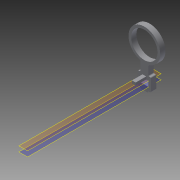
# Autodesk Inventor part: soporte-sujeccion-botella
Saved by Autodesk Inventor 2015 SP1 (Build 190203100, 203)
## iProperties
Created: 2015-07-19
Part Number: soporte-sujeccion-botella
Material: Genérico
Document SubType Name: Modeling
Designer: Javier
Density: 1 g/cm^3
Appearance: Valor por defecto
Author: Javier
Autodesk Inventor part; units mm, degrees
ref_plane "YZ Plane" through (0, 0, 0) normal (1, 0, 0) x (0, 1, 0)
ref_plane "XZ Plane" through (0, 0, 0) normal (0, 1, 0) x (-1, 0, 0)
ref_plane "XY Plane" through (0, 0, 0) normal (0, 0, 1) x (1, 0, 0)
ref_plane "Plano de trabajo1" through (0, 0, 0) normal (0, 0, 1) x (1, 0, 0)
sketch "Boceto1" plane through (0, 0, 0) normal (0, 0, 1) x (1, 0, 0)
  line L0 (9.5, 30) -> (9.5, 0) projected
  line L1 (9.5, 0) -> (15, 0) projected
  line L2 (15, 0) -> (15, 230) projected
  line L3 (0, 230) -> (15, 230) projected
  line L4 (0, 0) -> (0, 230) projected
  line L5 (0, 0) -> (5.5, 0) projected
  line L6 (5.5, 0) -> (5.5, 30) projected
  line L7 (9.5, 30) -> (5.5, 30) projected
  circle A0 centre (7.5, 223) radius 2 projected
  circle A1 centre (7.5, 213) radius 2 projected
  line L8 (0, 218) -> (15, 218)
  line L9 (15, 218) -> (15, 228)
  line L10 (15, 228) -> (0, 228)
  line L11 (0, 228) -> (0, 218)
  line L12 (0, 218) -> (15, 228) construction
  line L13 (15, 218) -> (0, 228) construction
  dimension "d0" = 10
  constraints: 12 end point, 2 midpoint, 2 parallel, 1 horizontal, 1 perpendicular, 1 point on line
  measures "d0" distance of L9.end L8.end
extrude "Extrusión1" add sketch "Boceto1" along normal blind 30 contours L8 L4 L10 L2 | A0
ref_plane "Plano de trabajo2" through (15, 0, -10) normal (0, 0, -1) x (-1, 0, 0)
sketch "Boceto2" plane through (15, 0, -10) normal (0, 0, -1) x (-1, 0, 0)
  line L0 (0, 228) -> (15, 228) projected
  line L1 (15, 228) -> (15, 218) projected
  line L2 (15, 218) -> (0, 218) projected
  line L3 (0, 218) -> (0, 228) projected
  circle A0 centre (7.5, 223) radius 2 projected
  point P0 (15, 0)
extrude "Extrusión2" add sketch "Boceto2" along normal blind 10
sketch "Boceto3" plane through (0, 218, 0) normal (0, -1, 0) x (1, 0, 0)
  line L0 (0, 0) -> (15, 0) projected
  line L1 (15, 0) -> (15, 30) projected
  line L2 (0, 30) -> (15, 30) projected
  line L3 (0, 0) -> (0, 30) projected
  line L4 (0, 0) -> (7.5, 0)
  line L5 (15, 0) -> (0, 0) projected
  line L6 (7.5, 0) -> (7.5, 2.5)
  line L7 (4, 5) -> (11, 5)
  line L8 (11, 5) -> (11, 0)
  line L9 (11, 0) -> (4, 0)
  line L10 (4, 0) -> (4, 5)
  line L11 (4, 5) -> (11, 0) construction
  line L12 (11, 5) -> (4, 0) construction
  dimension "d5" = 2.5
  dimension "d6" = 7
  dimension "d7" = 5
  constraints: 16 end point, 3 midpoint, 2 parallel, 2 perpendicular, 1 horizontal
  measures "d5" distance of L4.end L6.end
  measures "d6" distance of L8.end L9.end
  measures "d7" distance of L7.end L8.end
extrude "Extrusión3" add sketch "Boceto3" along normal blind 20 contours L10 L7 L8 L0
sketch "Boceto4" plane through (0, 218, -10) normal (0, -1, 0) x (1, 0, 0)
  line L0 (0, 0) -> (15, 0) projected
  line L1 (0, 0) -> (0, -10) projected
  line L2 (15, -10) -> (0, -10) projected
  line L3 (15, 0) -> (15, -10) projected
  line L4 (4, 10) -> (4, 15) projected
  line L5 (4, 15) -> (11, 15) projected
  line L6 (11, 15) -> (11, 10) projected
  line L7 (11, 10) -> (15, 10) projected
  line L8 (15, 10) -> (15, 40) projected
  line L9 (0, 40) -> (15, 40) projected
  line L10 (0, 10) -> (0, 40) projected
  line L11 (0, 10) -> (4, 10) projected
  line L12 (15, 10) -> (0, 10) projected
  line L13 (7.5, 10) -> (7.5, 0)
  line L14 (15, 0) -> (0, 0) projected
  line L15 (-5, 17.5) -> (20, 17.5)
  line L16 (20, 17.5) -> (20, -7.5)
  line L17 (20, -7.5) -> (-5, -7.5)
  line L18 (-5, -7.5) -> (-5, 17.5)
  line L19 (-5, 17.5) -> (20, -7.5) construction
  line L20 (20, 17.5) -> (-5, -7.5) construction
  line L21 (15, 0) -> (0, 0) projected
  line L22 (0, 0) -> (0, 10) projected
  line L23 (0, 10) -> (15, 10) projected
  line L24 (15, 10) -> (15, 0) projected
  point P0 (7.5, 5)
  dimension "d10" = 25
  dimension "d11" = 25
  constraints: 14 end point, 5 midpoint, 2 parallel, 1 horizontal, 1 perpendicular
  measures "d10" distance of L16.end L17.end
  measures "d11" distance of L15.end L16.end
extrude "Extrusión4" add sketch "Boceto4" against normal up to surface (10 mm away) contours L0 L3 L17 L1 | L1 L17 L18 L15 L10 L22 | L10 L15 L8 L7 L6 L5 L4 L11 | L24 L8 L15 L16 L17 L3 | L10 L9 L8 L15
fillet "Empalme1" radius 2 10 edges at (15, 223, -17.5) (15, 223, -20) (20, 223, -17.5) (0, 223, -20) (0, 223, -17.5) (-5, 223, -17.5) (-5, 223, 7.5) (0, 223, 7.5) (20, 223, 7.5) (15, 223, 7.5)
sketch "Boceto5" plane through (0, 228, 30) normal (0, 1, 0) x (1, 0, 0)
  line L0 (15, 0) -> (0, 0) projected
  line L1 (7.5, 0) -> (7.5, -25)
  line L2 (7.5, 0) -> (32.5, 0) construction
  circle A0 centre (7.5, -25) radius 25
  arc A1 (0, 4.0474) -> (15, 4.0474) centre (7.5, -25) ccw
  arc A2 (18, 22.5) -> (20, 24.5) centre (18, 24.5) ccw projected
  line L3 (20, 45.5) -> (20, 24.5) projected
  arc A3 (20, 45.5) -> (18, 47.5) centre (18, 45.5) ccw projected
  line L4 (16.7081, 47.5) -> (18, 47.5) projected
  arc A4 (14.854, 48.75) -> (16.7081, 47.5) centre (16.7081, 49.5) ccw projected
  arc A5 (14.854, 48.75) -> (13, 50) centre (13, 48) ccw projected
  line L5 (2, 50) -> (13, 50) projected
  arc A6 (2, 50) -> (0.146, 48.75) centre (2, 48) ccw projected
  arc A7 (-1.7081, 47.5) -> (0.146, 48.75) centre (-1.7081, 49.5) ccw projected
  line L6 (-3, 47.5) -> (-1.7081, 47.5) projected
  arc A8 (-3, 47.5) -> (-5, 45.5) centre (-3, 45.5) ccw projected
  line L7 (-5, 24.5) -> (-5, 45.5) projected
  arc A9 (-5, 24.5) -> (-3, 22.5) centre (-3, 24.5) ccw projected
  line L8 (-2, 22.5) -> (-3, 22.5) projected
  arc A10 (0, 20.5) -> (-2, 22.5) centre (-2, 20.5) ccw projected
  line L9 (0, 20.5) -> (0, 0) projected
  line L10 (15, 0) -> (0, 0) projected
  line L11 (15, 20.5) -> (15, 0) projected
  arc A11 (17, 22.5) -> (15, 20.5) centre (17, 20.5) ccw projected
  line L12 (18, 22.5) -> (17, 22.5) projected
  line L13 (15, 30) -> (15, 40) projected
  line L14 (15, 30) -> (0, 30) projected
  line L15 (0, 40) -> (0, 30) projected
  line L16 (15, 40) -> (0, 40) projected
  point P0 (0, 30)
  dimension "d15" = 25
  dimension "d16" = 90
  dimension "d17" = 60
  constraints: 4 end point, 2 coincident, 2 point on circle, 2 point on line, 1 centre point, 1 horizontal, 1 midpoint, 1 perpendicular, 1 vertical, 1 vertical alignment, 2 other
  measures "d15" distance of L1.start L1.end
  measures "d16" angle of L1 L2
  measures "d17" diameter of A1
extrude "Extrusión5" add sketch "Boceto5" against normal up to surface (10 mm away) contours L11 A1 L9 L0
fillet "Empalme2" radius 2 2 edges at (0, 223, 25.9526) (15, 223, 25.9526)
